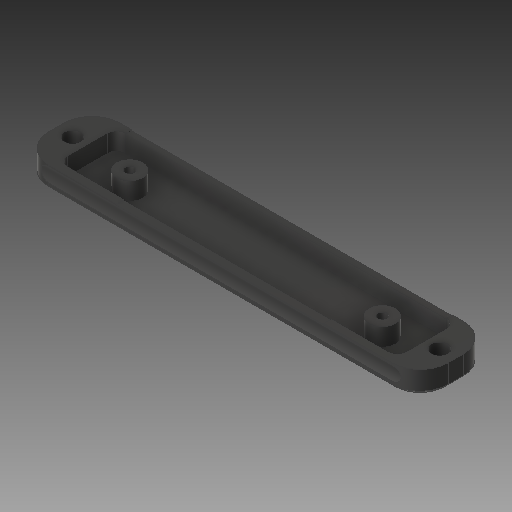
# Autodesk Inventor part: LR Top Cover Studs End
Saved by Autodesk Inventor 2019 (Build 230136000, 136)
## iProperties
Created: 2016-01-25
Part Number: LR Top Cover Studs End
Material: Acetal Resin, Black
Document SubType Name: Modeling
Designer: IEUser
Density: 1.425 g/cm^3
Appearance: Smooth - Black
Mass: 56.3375 g
Surface Area: 263.301 cm^2
Volume: 39.5351 cm^3
Author: IEUser
Autodesk Inventor part; units mm, degrees
ref_plane "YZ Plane" through (0, 0, 0) normal (1, 0, 0) x (0, 1, 0)
ref_plane "XZ Plane" through (0, 0, 0) normal (0, 1, 0) x (-1, 0, 0)
ref_plane "XY Plane" through (0, 0, 0) normal (0, 0, 1) x (1, 0, 0)
sketch "Body Outline" plane through (0, 0, 0) normal (0, 1, 0) x (-1, 0, 0)
  line L0 (106, -19) -> (-106, -19)
  line L1 (-106, -19) -> (-106, 19)
  line L2 (-106, 19) -> (106, 19)
  line L3 (106, 19) -> (106, -19)
  point P0 (0, 0)
  dimension "d0" = 38
  dimension "d1" = 19
  dimension "d2" = 212
  dimension "d3" = 106
  constraints: 8 end point, 2 parallel, 1 horizontal, 1 perpendicular
  measures "d0" distance of L0.end L1.end
  measures "d1" distance from line of point (0, 0) L0
  measures "d2" distance of L0.start L0.end
  measures "d3" distance from line of point (0, 0) L3
extrude "Body" add sketch "Body Outline" along normal blind 12
sketch "Body Cutout Outline" plane through (0, 12, 0) normal (0, 1, 0) x (1, 0, 0)
  line L0 (-90, -15) -> (90, -15)
  line L1 (90, -15) -> (90, 16)
  line L2 (90, 16) -> (-90, 16)
  line L3 (-90, 16) -> (-90, -15)
  circle A0 centre (-67, 0) radius 7
  circle A1 centre (67, 0) radius 7
  line L4 (-106, -19) -> (106, -19) projected
  point P0 (0, 0)
  dimension "d6" = 31
  dimension "d8" = 180
  dimension "d9" = 90
  dimension "d12" = 14
  dimension "d13" = 14
  dimension "d14" = 0
  dimension "d15" = 67
  dimension "d16" = 67
  dimension "d17" = 0
  dimension "d68" = 4
  constraints: 8 end point, 2 centre point, 2 parallel, 1 horizontal, 1 perpendicular
  measures "d6" distance of L2.end L0.start
  measures "d8" distance of L1.end L2.end
  measures "d9" distance from line of L1 point (0, 0)
  measures "d12" diameter of A0
  measures "d13" diameter of A1
  measures "d14" vertical distance of point (0, 0) A0.centre
  measures "d15" distance of point (0, 0) A0.centre
  measures "d16" distance of A1.centre point (0, 0)
  measures "d17" vertical distance of point (0, 0) A1.centre
  measures "d68" distance between parallel lines of L4 L0
extrude "Body Cutout" cut sketch "Body Cutout Outline" against normal blind 9.5
sketch "Skin Passages Outline" plane through (0, 12, 0) normal (0, 1, 0) x (1, 0, 0)
  line L0 (-85, 16) -> (85, 16)
  line L1 (85, 16) -> (85, 19)
  line L2 (85, 19) -> (-85, 19)
  line L3 (-85, 19) -> (-85, 16)
  line L4 (106, 19) -> (-106, 19) projected
  line L5 (-55, -19) -> (55, -19)
  line L6 (55, -19) -> (55, -15)
  line L7 (55, -15) -> (-55, -15)
  line L8 (-55, -15) -> (-55, -19)
  line L9 (-106, -19) -> (106, -19) projected
  point P0 (0, 0)
  dimension "d20" = 0
  dimension "d21" = 3
  dimension "d22" = 170
  dimension "d23" = 85
  dimension "d24" = 0
  dimension "d25" = 4
  dimension "d26" = 110
  dimension "d27" = 55
  constraints: 16 end point, 4 parallel, 2 horizontal, 2 perpendicular
  measures "d20" distance between parallel lines of L4 L2
  measures "d21" distance of L2.end L0.start
  measures "d22" distance of L1.end L2.end
  measures "d23" distance from line of point (0, 0) L3
  measures "d24" distance between parallel lines of L9 L5
  measures "d25" distance of L7.end L5.start
  measures "d26" distance of L5.start L5.end
  measures "d27" distance from line of point (0, 0) L8
extrude "Skin Passages" cut sketch "Skin Passages Outline" against normal blind 0.5
sketch "Fastening Hole Positions" plane through (0, 0, 0) normal (0, -1, 0) x (1, 0, 0)
  point P0 (0, 0)
  point P1 (67, 0)
  point P2 (-67, 0)
  dimension "d30" = 67
  dimension "d31" = 67
  dimension "d32" = 0
  dimension "d33" = 0
  measures "d30" distance of point (0, 0) point (67, 0)
  measures "d31" distance of point (0, 0) point (-67, 0)
  measures "d32" vertical distance of point (0, 0) point (67, 0)
  measures "d33" vertical distance of point (0, 0) point (-67, 0)
hole "Fastening Holes" at (67, 0, 0) at (-67, 0, 0) direction (0, 1, 0) diameter 5.1 end through all counterbore diameter 10.2 counterbore depth 7
sketch "Thumbscrew Hole Positions" plane through (0, 0, 0) normal (0, -1, 0) x (1, 0, 0)
  circle A0 centre (-97.35, 0) radius 4.5
  circle A1 centre (97.35, 0) radius 4.5
  line L0 (106, -19) -> (106, 19) projected
  line L1 (-106, 19) -> (-106, -19) projected
  point P0 (0, 0)
  dimension "d44" = 9
  dimension "d45" = 9
  dimension "d47" = 0
  dimension "d49" = 0
  dimension "d66" = 8.65
  dimension "d67" = 8.65
  constraints: 2 centre point
  measures "d44" diameter of A0
  measures "d45" diameter of A1
  measures "d47" vertical distance of point (0, 0) A0.centre
  measures "d49" vertical distance of point (0, 0) A1.centre
  measures "d66" distance from line of A1.centre L0
  measures "d67" distance from line of A0.centre L1
extrude "Thumbscrew Holes" cut sketch "Thumbscrew Hole Positions" along normal through all both and the other way through all
sketch "Side Cutout Outline" plane through (-106, 0, -19) normal (-1, 0, 0) x (0, 0, 1)
  circle A0 centre (47.3, 7.25) radius 10
  line L0 (38, 0) -> (38, 12) projected
  line L1 (0, 12) -> (38, 12) projected
  point P0 (19, 0)
  dimension "d69" = 20
  dimension "d70" = 9.3
  dimension "d71" = 4.75
  constraints: 1 centre point
  measures "d69" diameter of A0
  measures "d70" distance from line of A0.centre L0
  measures "d71" distance from line of A0.centre L1
extrude "Side Cutout" cut sketch "Side Cutout Outline" along normal through all both and the other way through all
fillet "Body Fillet" radius 5 4 edges at (-90, 7.25, -16) (90, 7.25, -16) (90, 7.25, 15) (-90, 7.25, 15)
fillet "Body Fillet" radius 15 4 edges at (-106, 1.7872, 19) (-106, 6, -19) (106, 6, -19) (106, 1.7872, 19)
chamfer "Body Chamfer" distance 2 angle 45 4 edges at (0, 0, 19) (106, 0, 0) (0, 0, -19) (-106, 0, 0)
equation "\"d1\" = 0.5 * d0"
equation "\"d3\" = 0.5 * d2"
equation "\"d9\" = 0.5 * d8"
equation "\"d16\" = d15"
equation "\"d23\" = 0.5 * d22"
equation "\"d27\" = 0.5 * d26"
body "Solid1"
